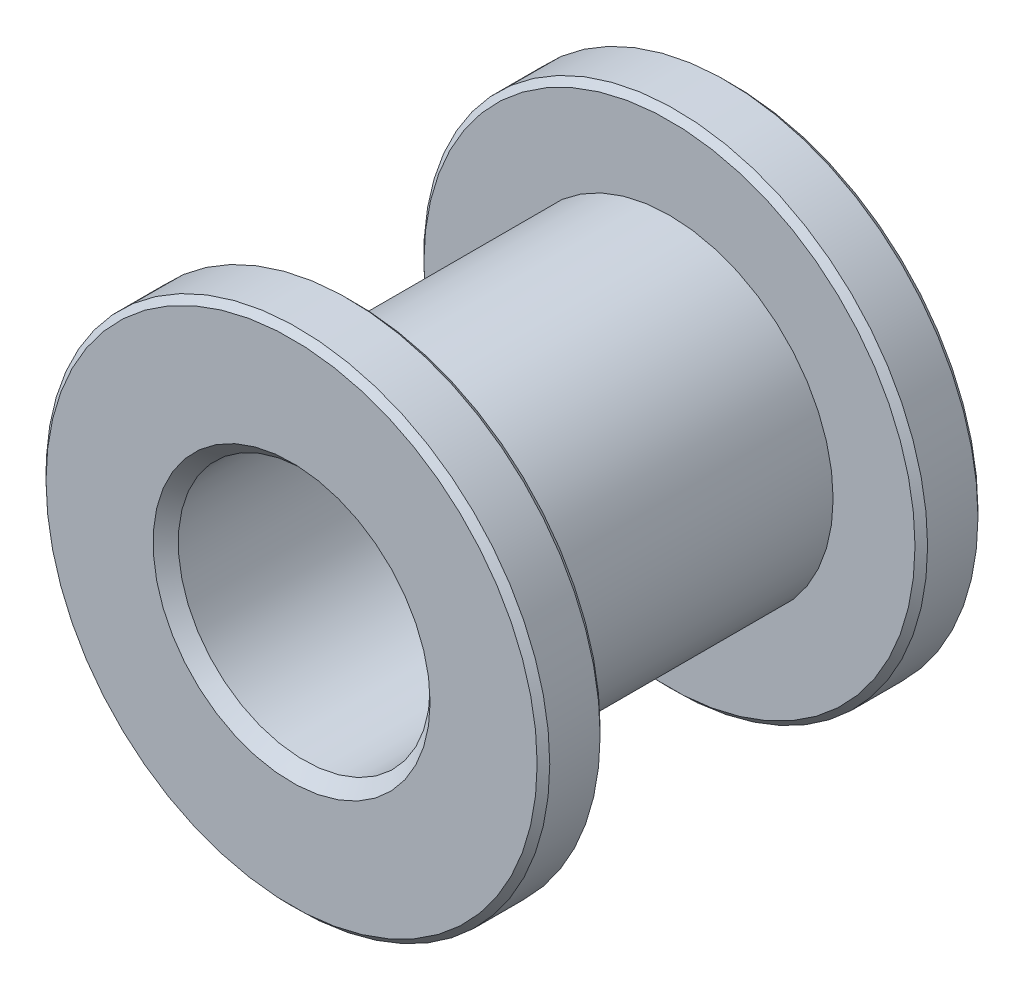
# Autodesk Inventor part: Holkki
Saved by Autodesk Inventor 2014 (Build 180170000, 170)
## iProperties
Created: 2013-09-01
Part Number: Holkki
Material: Polyethylene, High Density
Document SubType Name: Modeling
Designer: Arto
Density: 0.952 g/cm^3
Appearance: Blanche
Author: Arto
Autodesk Inventor part; units mm, degrees
ref_plane "YZ Plane" through (0, 0, 0) normal (1, 0, 0) x (0, 1, 0)
ref_plane "XZ Plane" through (0, 0, 0) normal (0, 1, 0) x (-1, 0, 0)
ref_plane "XY Plane" through (0, 0, 0) normal (0, 0, 1) x (1, 0, 0)
sketch "Sketch1" plane through (0, 0, 0) normal (0, 0, 1) x (1, 0, 0)
  circle A0 centre (27.2718, 25) radius 13 projected
  circle A1 centre (27.2718, 25) radius 10
  point P0 (0, 0)
  dimension "d0" = 20
  constraints: 1 centre point, 1 coincident
  measures "d0" diameter of A1
extrude "Extrusion1" add sketch "Sketch1" against normal blind 12.5
sketch "Sketch2" plane through (27.2718, 25, 0) normal (0, 0, 1) x (1, 0, 0)
  circle A0 centre (0, 0) radius 20
  circle A1 centre (0, 0) radius 10 projected
  point P0 (-27.2718, -25)
  dimension "d4" = 40
  constraints: 1 centre point
  measures "d4" diameter of A0
extrude "Extrusion2" add sketch "Sketch2" along normal blind 5
mirror "Mirror1" about plane through (27.2718, 25, -12.5) normal (0, 0, -1) of "Extrusion1", "Extrusion2"
chamfer "Chamfer1" distance 0.5 angle 45 4 edges at (7.2718, 25, -30) (7.2718, 25, 5) (7.2718, 25, 0) (7.2718, 25, -25)
chamfer "Chamfer2" distance 1 angle 45 2 edges at (17.2718, 25, 5) (17.2718, 25, -30)
body "Solid1"
